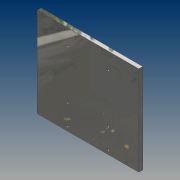
# Autodesk Inventor part: 08_Tam_truc_Z
Saved by Autodesk Inventor 2021 (Build 250183000, 183)
## iProperties
Created: 2024-04-08
Part Number: 08_Tam_truc_Z
Material: Stainless Steel, Austenitic
Document SubType Name: Modeling
Designer: Admin
Density: 8 g/cm^3
Appearance: Semi-Polished
Mass: 4400 g
Surface Area: 1194 cm^2
Volume: 550 cm^3
Author: Admin
Autodesk Inventor part; units mm, degrees
ref_plane "YZ Plane" through (0, 0, 0) normal (1, 0, 0) x (0, 1, 0)
ref_plane "XZ Plane" through (0, 0, 0) normal (0, 1, 0) x (-1, 0, 0)
ref_plane "XY Plane" through (0, 0, 0) normal (0, 0, 1) x (1, 0, 0)
sketch "Sketch1" plane through (0, 0, 0) normal (0, 0, 1) x (1, 0, 0)
  line L0 (-125, -110) -> (-125, 110)
  line L1 (-125, 110) -> (125, 110)
  line L2 (125, 110) -> (125, -110)
  line L3 (125, -110) -> (-125, -110)
  line L4 (-125, -110) -> (125, 110) construction
  line L5 (-125, 110) -> (125, -110) construction
  point P0 (0, 0)
  dimension "d0" = 220
  dimension "d1" = 250
  constraints: 12 end point, 2 midpoint, 2 parallel, 1 perpendicular, 1 vertical
  measures "d0" distance of L1.end L2.end
  measures "d1" distance between parallel lines of L0 L2
extrude "Extrusion1" add sketch "Sketch1" along normal blind 10
sketch "Sketch2" plane through (0, 0, 0) normal (0, 0, -1) x (-1, 0, 0)
  line L0 (50, 100) -> (-50, 100)
  line L1 (-50, 100) -> (-50, -100)
  line L2 (-50, -100) -> (50, -100)
  line L3 (50, -100) -> (50, 100)
  line L4 (50, 100) -> (-50, -100) construction
  line L5 (-50, 100) -> (50, -100) construction
  line L6 (-125, -110) -> (-125, 110) projected
  line L7 (125, -110) -> (-125, -110) projected
  point P0 (0, 0)
  point P1 (50, -50)
  point P2 (50, 70)
  point P3 (-50, -50)
  point P4 (-50, 70)
  dimension "d4" = 75
  dimension "d5" = 10
  dimension "d6" = 50
  dimension "d7" = 30
  constraints: 12 end point, 4 point on line, 2 coincident, 2 horizontal alignment, 2 midpoint, 2 parallel, 1 horizontal, 1 perpendicular
  measures "d4" distance between parallel lines of L6 L1
  measures "d5" distance between parallel lines of L7 L2
  measures "d6" distance from line of L2 point (-50, -50)
  measures "d7" distance from line of L0 point (-50, 70)
hole "Hole1" at (-50, -50, 0) at (-50, 70, 0) at (50, -50, 0) at (50, 70, 0) at (50, -100, 0) at (-50, -100, 0) direction (0, 0, 1) diameter 4.5 end through all
sketch "Sketch3" plane through (0, 0, 10) normal (0, 0, 1) x (1, 0, 0)
  line L0 (109.42, -76) -> (119.92, -76) projected
  line L1 (109.42, -76) -> (109.42, -90) projected
  line L2 (109.42, -90) -> (119.92, -90) projected
  line L3 (119.92, -90) -> (119.92, -76) projected
  circle A0 centre (115.92, -83) radius 3 projected
  line L4 (79.92, -90) -> (90.42, -90) projected
  line L5 (90.42, -90) -> (90.42, -76) projected
  line L6 (79.92, -76) -> (90.42, -76) projected
  line L7 (79.92, -76) -> (79.92, -90) projected
  circle A1 centre (83.92, -83) radius 3 projected
  line L8 (34, -69) -> (34, -93) projected
  line L9 (18, -69) -> (34, -69) projected
  line L10 (18, -93) -> (18, -69) projected
  line L11 (34, -93) -> (18, -93) projected
  circle A2 centre (26.5, -81) radius 5 projected
  circle A3 centre (-26.5, -81) radius 5 projected
  line L12 (-34, -93) -> (-34, -69) projected
  line L13 (-18, -93) -> (-34, -93) projected
  line L14 (-18, -93) -> (-18, -69) projected
  line L15 (-34, -69) -> (-18, -69) projected
  circle A4 centre (-26.5, -81) radius 5 projected
  line L16 (-79.92, -76) -> (-90.42, -76) projected
  line L17 (-90.42, -76) -> (-90.42, -90) projected
  line L18 (-79.92, -90) -> (-90.42, -90) projected
  line L19 (-79.92, -90) -> (-79.92, -76) projected
  circle A5 centre (-83.92, -83) radius 3 projected
  line L20 (-109.42, -90) -> (-119.92, -90) projected
  line L21 (-109.42, -90) -> (-109.42, -76) projected
  line L22 (-109.42, -76) -> (-119.92, -76) projected
  line L23 (-119.92, -76) -> (-119.92, -90) projected
  circle A6 centre (-115.92, -83) radius 3 projected
  line L24 (-34, 70) -> (-34, 90) projected
  line L25 (-18, 70) -> (-34, 70) projected
  line L26 (-18, 90) -> (-18, 70) projected
  line L27 (-34, 90) -> (-18, 90) projected
  circle A7 centre (-26.5, 80) radius 4.5 projected
  line L28 (34, 90) -> (34, 70) projected
  line L29 (18, 90) -> (34, 90) projected
  line L30 (18, 90) -> (18, 70) projected
  line L31 (34, 70) -> (18, 70) projected
  circle A8 centre (26.5, 80) radius 4.5 projected
  point P0 (0, 0)
extrude "Extrusion2" cut sketch "Sketch3" against normal blind 10 contours A0 | A1 | A2 | A3 | A5 | A6 | A7 | A8
body "Solid1"
